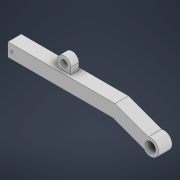
# Autodesk Inventor part: Fahrwerk_rocker_hinten
Saved by Autodesk Inventor 2021 (Build 250183000, 183)
## iProperties
Created: 2020-12-28
Part Number: Fahrwerk_rocker_hinten
Material: Generisch
Document SubType Name: Modeling
Designer: laure
Density: 1 g/cm^3
Appearance: Vorgabe
Author: laure
Autodesk Inventor part; units mm, degrees
ref_plane "YZ Plane" through (0, 0, 0) normal (1, 0, 0) x (0, 1, 0)
ref_plane "XZ Plane" through (0, 0, 0) normal (0, 1, 0) x (-1, 0, 0)
ref_plane "XY Plane" through (0, 0, 0) normal (0, 0, 1) x (1, 0, 0)
sketch "Skizze1" plane through (0, 0, 0) normal (0, 0, 1) x (1, 0, 0)
  line L0 (-110, 10) -> (50, 10)
  line L1 (46.4735, -10) -> (-110, -10)
  line L2 (-153.2763, 0) -> (149.6579, 0) projected
  line L3 (99.5412, -29.3151) -> (46.4735, -10)
  line L4 (50, 10) -> (106.3816, -10.5212)
  line L5 (106.3816, -10.5212) -> (99.5412, -29.3151)
  line L6 (0, -37.1781) -> (0, 17.863) projected
  line L7 (-110, 10) -> (-110, -10)
  point P0 (0, 0)
  dimension "d5" = 20
  dimension "d56" = 0
  dimension "d57" = 0
  dimension "d58" = 60
  dimension "d138" = 160
  dimension "d140" = 20
  dimension "d141" = 10
  dimension "d142" = 110
  dimension "d143" = 50
  dimension "d144" = 10
  constraints: 12 end point, 2 parallel, 2 perpendicular, 1 horizontal, 1 other
  measures "d5" distance between parallel lines of L4 L3
  measures "d56" distance from line of L0 L4.start
  measures "d57" distance of L0.end L4.start
  measures "d58" distance from line of L4.start L5
  measures "d138" distance from line of L7 L0.end
  measures "d140" angle of L6 L5
  measures "d141" distance between parallel lines of L2 L0
  measures "d142" distance between parallel lines of L6 L7
  measures "d143" distance from line of point (50, 10) L6
  measures "d144" distance from line of point (50, 10) L2
sketch "Skizze4" plane through (0, 0, 0) normal (0, 0, 1) x (1, 0, 0)
  line L0 (-40, 10) -> (-20, 10)
  line L1 (-20, 10) -> (-20, 20)
  line L2 (-30, 30) -> (-30, 30)
  line L3 (-40, 20) -> (-40, 10)
  circle A0 centre (-30, 20) radius 4.875
  arc A1 (-30, 30) -> (-40, 20) centre (-30, 20) ccw
  arc A2 (-20, 20) -> (-30, 30) centre (-30, 20) ccw
  line L4 (-50.4853, 0) -> (8.4142, 0) projected
  line L5 (0, -6.4142) -> (0, 38.4853) projected
  point P0 (0, 0)
  point P1 (-30, 30)
  dimension "d74" = 20
  dimension "d75" = 20
  dimension "d76" = 9.75
  dimension "d77" = 10
  dimension "d78" = 10
  dimension "d115" = 10
  dimension "d116" = 10
  dimension "d139" = 30
  constraints: 8 end point, 4 point on circle, 4 tangent, 3 centre point, 2 parallel, 1 concentric, 1 horizontal, 1 perpendicular
  measures "d74" distance between parallel lines of L1 L3
  measures "d75" distance between parallel lines of L0 L2
  measures "d76" diameter of A0
  measures "d77" distance from line of A0.centre L0
  measures "d78" radius of A1
  measures "d115" distance from line of L3 A0.centre
  measures "d116" distance between parallel lines of L0 L4
  measures "d139" distance from line of L5 A0.centre
extrude "Extrusion1" add sketch "Skizze1" against normal mid plane 20
sketch "Skizze13" plane through (0, 0, -10) normal (0, 0, -1) x (-1, 0, 0)
  line L0 (-106.3816, -10.5212) -> (-99.5412, -29.3151) projected
  circle A0 centre (-102.9614, -19.9181) radius 7.65
  circle A1 centre (-102.9614, -19.9181) radius 12.25
  point P0 (0, 0)
  point P1 (-105.5778, -12.7295)
  point P2 (-100.3449, -27.1068)
  dimension "d148" = 15.3
  dimension "d149" = 24.5
  constraints: 2 centre point, 1 coincident, 1 midpoint
  measures "d148" diameter of A0
  measures "d149" diameter of A1
extrude "Extrusion13" add sketch "Skizze13" against normal blind 20
extrude "Extrusion14" cut sketch "Skizze13" against normal up to surface (20 mm away) contours A0 L0 picked at (-100.4872, -20.535)
shell "Wandung2" thickness 2.6 removed faces 1 at (-110, -3.3333, -3.3333)
extrude "Extrusion11" add sketch "Skizze4" against normal mid plane 12
sketch "Skizze12" plane through (0, 0, 10) normal (0, 0, 1) x (1, 0, 0)
  circle A0 centre (-104, 0) radius 1.6
  line L0 (-110, 6) -> (49.2947, 6) projected
  line L1 (-110, 10) -> (-110, -10) projected
  line L2 (50, 10) -> (-110, 10) projected
  point P0 (0, 0)
  point P1 (-110, -6)
  dimension "d133" = 3.2
  dimension "d135" = 6
  dimension "d147" = 10
  constraints: 1 centre point
  measures "d133" diameter of A0
  measures "d135" distance from line of L1 A0.centre
  measures "d147" distance from line of A0.centre L2
extrude "Extrusion12" cut sketch "Skizze12" against normal up to surface (20 mm away)
